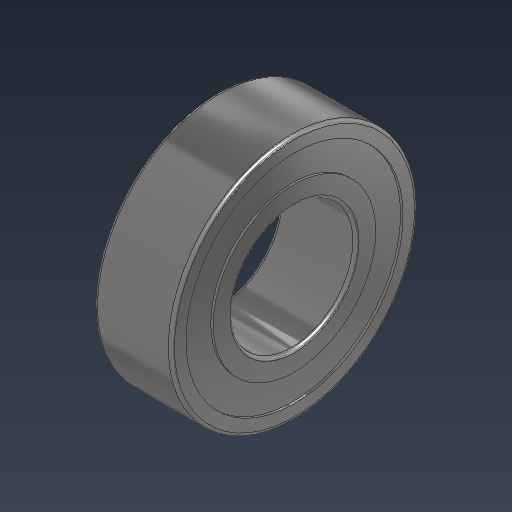
# Autodesk Inventor part: B688ZZ
Saved by Autodesk Inventor 2021 (Build 250183000, 183)
## iProperties
Category: PARTsolutions
Company: MISUMI
Part Number: B688ZZ
Material: 鋼、合金
Catalog Web Link: www.cadenas.de
Description: B6 _ _ ZZ, B6 _ _ AZZ, SB6 _ _ ZZ, SB6 _ _ AZZ, BR _ _ ZZ, SBR _ _ ZZ-Small Ball Bearings - Double Shield Type
Vendor: MISUMI
Document SubType Name: Modeling
Designer: partserver
Manufacturer: MISUMI
Mass: 5.64802 g
Surface Area: 6.90443 cm^2
Volume: 0.730663 cm^3
Density: 7.73 g/cm^3
Appearance: 半つや出し
PSOL_IDENT_0: {$CADENAS_DATA\23d-libs\misumi\metric\12_bearing_holders\sb685zz.prj},219 {VTYP=3D},{NB=B688ZZ},{LIN
PSOL_IDENT_1: A=B688ZZ},{NN=B6 _ _ ZZ, B6 _ _ AZZ, SB6 _ _ ZZ, SB6 _ _ AZZ, BR _ _ ZZ, SBR _ _ ZZ},{DATE=09.09.201
PSOL_IDENT_2: 9 15:26:56},{GEOMDATE=23.07.2013 00:00:00},{VERSION=},{LINEID=270},{WBVAR=MAT},{WBNUMERIC=}  {NB=B68
PSOL_IDENT_3: 8ZZ},{LINA=B688ZZ},{KT=DUMMY},{PN=B688ZZ},{MAT=},{BN=688ZZ},{DD=8.0},{A=4.6800},{BB=0.944},{C=1.280}
PSOL_IDENT_4: ,{D=16},{B=5.0},{RR=0.20},{CR=1610},{COR=715},{CRS=1610},{CRSS=1368},{CORS=715},{CORSS=572},{DS=9.60
PSOL_IDENT_5: },{DDHH=14.40},{R=0.20},{MASS=4.02},{X=0},{BN2=B688ZZ}
NB: B688ZZ
NN: B6 _ _ ZZ, B6 _ _ AZZ, SB6 _ _ ZZ, SB6 _ _ AZZ, BR _ _ ZZ, SBR _ _ ZZ
NT: Small Ball Bearings - Double Shield Type
NBSYN: $PN.
LINA: B688ZZ
CATALOG: Misumi
PN: B688ZZ
MAT: 52100 Bearing Steel
BN: 688ZZ
DD: 8
D: 16
B: 5
RR: 0.2
CR: 1610
COR: 715
DS: 9.6
DDHH: 14.4
R: 0.2
MASS: 4.02
X: 0
SUPPLIER: MISUMI
ARTICLENO: B688ZZ
BOMINFO: B688ZZ
CREATOR: CADENAS GmbH
購入先: ミスミ
在庫数: 0.0
状態: 688ZZ
代替品型番: 688ZZ
Title: B688ZZ
Author: Cadenas PARTsolutions
Comments: Small Ball Bearings - Double Shield Type
Autodesk Inventor part; units mm, degrees
sketch "Sketch_1" plane through (0, 0, 0) normal (0, 0, 1) x (1, 0, 0)
  line L0 (4.8, 0) -> (0.2, 0)
  arc A0 (0, 4.2) -> (0.2, 4) centre (0.2, 4.2) ccw
  line L1 (0.2, 4) -> (4.8, 4)
  arc A1 (4.8, 4) -> (5, 4.2) centre (4.8, 4.2) ccw
  line L2 (5, 4.2) -> (5, 5.28)
  line L3 (5, 5.28) -> (4.84, 5.28)
  line L4 (4.84, 5.28) -> (4.84, 7.056)
  line L5 (4.84, 7.056) -> (5, 7.056)
  line L6 (5, 7.056) -> (5, 7.8)
  arc A2 (5, 7.8) -> (4.8, 8) centre (4.8, 7.8) ccw
  line L7 (4.8, 8) -> (0.2, 8)
  arc A3 (0.2, 8) -> (0, 7.8) centre (0.2, 7.8) ccw
  line L8 (0, 7.8) -> (0, 7.056)
  line L9 (0, 7.056) -> (0.16, 7.056)
  line L10 (0.16, 7.056) -> (0.16, 5.28)
  line L11 (0.16, 5.28) -> (0, 5.28)
  line L12 (0, 5.28) -> (0, 4.2)
  constraints: 26 end point, 8 point on circle, 4 centre point
revolve "Revolution1" add sketch "Sketch_1" angle 360 about axis through (4.8, 0, 0) along (1, 0, 0)
ref_plane "to_housing_XY" through (0, 0, 0) normal (1, 0, 0) x (0, 0, -1)
ref_plane "to_housing_YZ" through (0, 0, 0) normal (0, 0, -1) x (0, 1, 0)
ref_plane "to_housing_ZX" through (0, 0, 0) normal (0, 1, 0) x (1, 0, 0)
ref_plane "to_housing_center_XY" through (2.5, 0, 0) normal (1, 0, 0) x (0, 0, -1)
ref_plane "to_housing_center_YZ" through (2.5, 0, 0) normal (0, 0, -1) x (0, 1, 0)
ref_plane "to_housing_center_ZX" through (2.5, 0, 0) normal (0, 1, 0) x (1, 0, 0)
body "Solid1"
